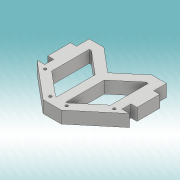
# Autodesk Inventor part: Leg_part2
Saved by Autodesk Inventor 2019 (Build 230136000, 136)
## iProperties
Created: 2019-01-31
Part Number: Leg_part2
Material: Generic
Document SubType Name: Modeling
Designer: nelson.soberon
Density: 1 g/cm^3
Appearance: Default
Author: nelson.soberon
Autodesk Inventor part; units mm, degrees
ref_plane "YZ Plane" through (0, 0, 0) normal (1, 0, 0) x (0, 1, 0)
ref_plane "XZ Plane" through (0, 0, 0) normal (0, 1, 0) x (-1, 0, 0)
ref_plane "XY Plane" through (0, 0, 0) normal (0, 0, 1) x (1, 0, 0)
sketch "Sketch1" plane through (0, 0, 0) normal (0, 0, 1) x (1, 0, 0)
  line L0 (0, 0) -> (-6, 0)
  line L1 (-6, 0) -> (-30.5134, 20.5692)
  line L2 (-19.5134, 44) -> (-19.5134, 19.1716)
  line L3 (-19.5134, 19.1716) -> (-3.8162, 6)
  line L4 (0, 0) -> (0, 7.1987)
  circle A0 centre (-5.4048, 4.2) radius 0.889
  circle A1 centre (-22.8134, 18.1692) radius 0.889
  line L5 (-30.5134, 20.5692) -> (-25.4999, 20.5692)
  line L6 (-25.4999, 20.5692) -> (-25.4999, 26.5692)
  line L7 (-25.4999, 26.5692) -> (-29.4999, 26.5692)
  line L8 (-29.4999, 26.5692) -> (-29.4999, 41.5692)
  line L9 (-29.4999, 41.5692) -> (-25.4999, 41.5692)
  line L10 (-25.4999, 41.5692) -> (-25.4999, 50)
  line L11 (-25.4999, 50) -> (-15.8296, 50)
  line L12 (-15.8296, 50) -> (0, 36.7174)
  line L13 (-3, 31.4022) -> (-3, 6)
  line L14 (0, 7.1987) -> (0, 36.7174)
  line L15 (-18.0134, 44) -> (-3, 31.4022)
  line L16 (-19.5134, 44) -> (-18.0134, 44)
  line L17 (-3.8162, 6) -> (-3, 6)
  line L18 (0, 0) -> (6, 0)
  circle A2 centre (5.4048, 4.2) radius 0.889
  line L19 (19.5134, 19.1716) -> (3.8162, 6)
  line L20 (19.5134, 44) -> (19.5134, 19.1716)
  line L21 (6, 0) -> (30.5134, 20.5692)
  circle A3 centre (22.8134, 18.1692) radius 0.889
  line L22 (30.5134, 20.5692) -> (25.4999, 20.5692)
  line L23 (25.4999, 20.5692) -> (25.4999, 26.5692)
  line L24 (25.4999, 26.5692) -> (29.4999, 26.5692)
  line L25 (29.4999, 26.5692) -> (29.4999, 41.5692)
  line L26 (29.4999, 41.5692) -> (25.4999, 41.5692)
  line L27 (25.4999, 41.5692) -> (25.4999, 50)
  line L28 (25.4999, 50) -> (15.8296, 50)
  line L29 (15.8296, 50) -> (0, 36.7174)
  line L30 (3, 31.4022) -> (3, 6)
  line L31 (18.0134, 44) -> (3, 31.4022)
  line L32 (19.5134, 44) -> (18.0134, 44)
  line L33 (3.8162, 6) -> (3, 6)
  dimension "d0" = 6
  dimension "d2" = 40
  dimension "d5" = 1.778
  dimension "d6" = 32
  dimension "d8" = 3.3
  dimension "d9" = 2.4
  dimension "d10" = 4.2
  dimension "d11" = 6
  dimension "d13" = 5.0135
  dimension "d14" = 2.4
  dimension "d21" = 6
  dimension "d22" = 6
  dimension "d23" = 1.5
  dimension "d24" = 15
  dimension "d25" = 4
  dimension "d30" = 6
  dimension "d32" = 6
  dimension "d33" = 6
  dimension "d34" = 5.9865
  dimension "d35" = 50
  constraints: 70 end point, 17 symmetric about line, 5 horizontal, 5 vertical, 4 centre point, 4 parallel, 4 perpendicular, 1 coincident, 1 equal radius, 2 other
  measures "d0" distance of L4.start L0.end
  measures "d2" angle of L0 L1
  measures "d5" diameter of A0
  measures "d6" distance of L0.end L1.end
  measures "d8" distance from line of A1.centre L2
  measures "d9" distance from line of L3 A0.centre
  measures "d10" distance from line of L0 A0.centre
  measures "d11" distance between parallel lines of L3 L1
  measures "d13" distance of L1.end L5.end
  measures "d14" distance from line of L5 A1.centre
  measures "d21" distance between parallel lines of L12 L15
  measures "d22" distance between parallel lines of L11 L16
  measures "d23" distance of L2.start L15.start
  measures "d24" distance of L7.end L8.end
  measures "d25" distance of L8.end L9.end
  measures "d30" distance between parallel lines of L0 L17
  measures "d32" diameter of L13 L14
  measures "d33" distance of L5.end L6.end
  measures "d34" distance between parallel lines of L2 L6
  measures "d35" distance between parallel lines of L0 L11
extrude "Extrusion1" add sketch "Sketch1" along normal mid plane 8
body "Solid1"
